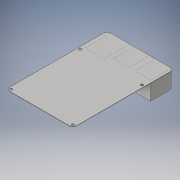
# Autodesk Inventor part: RPI
Saved by Autodesk Inventor 2016 (Build 200138000, 138)
## iProperties
Created: 2017-10-12
Part Number: RPI
Material: Generic
Document SubType Name: Modeling
Designer: Student
Density: 1 g/cm^3
Appearance: Default
Author: Student
Autodesk Inventor part; units mm, degrees
ref_plane "YZ Plane" through (0, 0, 0) normal (1, 0, 0) x (0, 1, 0)
ref_plane "XZ Plane" through (0, 0, 0) normal (0, 1, 0) x (-1, 0, 0)
ref_plane "XY Plane" through (0, 0, 0) normal (0, 0, 1) x (1, 0, 0)
sketch "Sketch1" plane through (0, 0, 0) normal (0, 1, 0) x (-1, 0, 0)
  line L0 (28.4786, 33.7956) -> (-27.6046, 33.7956)
  line L1 (-27.6046, 33.7956) -> (-27.6046, -50.9896)
  line L2 (-27.6046, -50.9896) -> (28.4786, -50.9896)
  line L3 (28.4786, -50.9896) -> (28.4786, 33.7956)
  point P0 (0, 0)
  dimension "d0" = 56.0832
  dimension "d1" = 84.7852
  constraints: 8 end point, 2 parallel, 1 horizontal, 1 perpendicular
  measures "d0" distance of L0.start L0.end
  measures "d1" distance of L2.end L0.start
extrude "Extrusion1" add sketch "Sketch1" along normal blind 0.1956
fillet "Fillet1" radius 3.175 4 edges at (27.6046, 0.0978, -50.9896) (-28.4786, 0.0978, -50.9896) (-28.4786, 0.0978, 33.7956) (27.6046, 0.0978, 33.7956)
sketch "Sketch2" plane through (0, 0, 0) normal (0, -1, 0) x (1, 0, 0)
  line L0 (-28.4786, -47.8146) -> (-28.4786, 30.6206) construction
  line L1 (-28.4786, 31.6112) -> (-26.2942, 31.6112) construction
  line L2 (-26.2942, 31.6112) -> (-26.2942, 33.7956) construction
  line L3 (-25.3036, 33.7956) -> (24.4296, 33.7956) construction
  circle A0 centre (-26.2942, 31.6112) radius 1.0922
  line L4 (27.6046, 30.6206) -> (27.6046, -47.8146) construction
  line L5 (27.6046, 31.6112) -> (25.4202, 31.6112) construction
  line L6 (25.4202, 31.6112) -> (25.4202, 33.7956) construction
  circle A1 centre (25.4202, 31.6112) radius 1.0922
  circle A2 centre (-26.2942, -26.3261) radius 1.0921
  circle A3 centre (25.4202, -26.3261) radius 1.0921
  point P0 (0, 0)
  dimension "d5" = 2.1844
  dimension "d6" = 2.1844
  dimension "d7" = 2.1844
  dimension "d8" = 2.1844
  dimension "d9" = 55.753
  dimension "d10" = 55.753
  constraints: 8 end point, 4 centre point, 4 point on line, 2 coincident, 2 horizontal, 2 perpendicular
  measures "d5" distance between parallel lines of L3 L1
  measures "d6" distance between parallel lines of L0 L2
  measures "d7" distance between parallel lines of L4 L6
  measures "d8" distance between parallel lines of L3 L5
extrude "Extrusion2" cut sketch "Sketch2" against normal blind 0.1956
sketch "Sketch3" plane through (0, 0, 0) normal (0, -1, 0) x (1, 0, 0)
  line L0 (25.4202, -33.5906) -> (12.0344, -33.5906)
  line L1 (12.0344, -33.5906) -> (12.0344, -50.9896)
  line L2 (12.0344, -50.9896) -> (25.4202, -50.9896)
  line L3 (25.4202, -50.9896) -> (25.4202, -33.5906)
  line L4 (7.3354, -33.5906) -> (-6.0504, -33.5906)
  line L5 (-6.0504, -33.5906) -> (-6.0504, -50.9896)
  line L6 (-6.0504, -50.9896) -> (7.3354, -50.9896)
  line L7 (7.3354, -50.9896) -> (7.3354, -33.5906)
  line L8 (-25.5576, -29.7298) -> (-9.6318, -29.7298)
  line L9 (-9.6318, -29.7298) -> (-9.6318, -50.9896)
  line L10 (-9.6318, -50.9896) -> (-25.5576, -50.9896)
  line L11 (-25.5576, -50.9896) -> (-25.5576, -29.7298)
  line L12 (24.4296, -50.9896) -> (-25.3036, -50.9896) projected
  line L13 (27.6046, 30.6206) -> (27.6046, -47.8146) projected
  point P0 (0, 0)
  dimension "d13" = 13.3858
  dimension "d14" = 13.3858
  dimension "d16" = 17.399
  dimension "d18" = 21.2598
  dimension "d19" = 15.9258
  dimension "d20" = 0
  dimension "d21" = 0
  dimension "d22" = 4.699
  dimension "d23" = 3.5814
  dimension "d24" = 2.1844
  constraints: 24 end point, 6 parallel, 3 horizontal, 3 perpendicular, 2 point on line
  measures "d13" distance of L0.start L0.end
  measures "d14" distance of L4.start L4.end
  measures "d16" distance of L2.end L0.start
  measures "d18" distance of L8.end L9.end
  measures "d19" distance of L8.start L8.end
  measures "d20" distance between parallel lines of L12 L2
  measures "d21" distance between parallel lines of L12 L10
  measures "d22" distance between parallel lines of L7 L1
  measures "d23" distance between parallel lines of L9 L5
  measures "d24" distance between parallel lines of L3 L13
extrude "Extrusion3" add sketch "Sketch3" along normal blind 15.24
equation "\"d6\" = d5"
equation "\"d7\" = d6"
equation "\"d8\" = d5"
equation "\"d10\" = d9"
equation "\"d14\" = d13"
body "Solid1"
